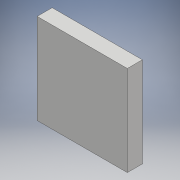
# Autodesk Inventor part: example_sample
Saved by Autodesk Inventor 2017 (Build 210142000, 142)
## iProperties
Created: 2018-01-08
Part Number: example_sample
Material: Generic
Document SubType Name: Modeling
Designer: Sam
Density: 1 g/cm^3
Appearance: Default
Author: Sam
Autodesk Inventor part; units mm, degrees
ref_plane "YZ Plane" through (0, 0, 0) normal (1, 0, 0) x (0, 1, 0)
ref_plane "XZ Plane" through (0, 0, 0) normal (0, 1, 0) x (-1, 0, 0)
ref_plane "XY Plane" through (0, 0, 0) normal (0, 0, 1) x (1, 0, 0)
sketch "Sketch1" plane through (0, 0, 0) normal (0, 1, 0) x (-1, 0, 0)
  line L0 (6, 6) -> (-6, 6)
  line L1 (-6, 6) -> (-6, -6)
  line L2 (-6, -6) -> (6, -6)
  line L3 (6, -6) -> (6, 6)
  line L4 (6, 6) -> (-6, -6) construction
  line L5 (-6, 6) -> (6, -6) construction
  point P0 (0, 0)
  dimension "d0" = 12
  dimension "d1" = 12
  constraints: 12 end point, 2 midpoint, 2 parallel, 1 horizontal, 1 perpendicular
  measures "d0" distance of L2.end L1.end
  measures "d1" distance of L1.end L0.end
extrude "Extrusion1" add sketch "Sketch1" along normal blind 2
sketch "Sketch2" plane through (0, 2, 0) normal (0, 1, 0) x (1, 0, 0)
  line L0 (-0.0927, -0.2032) -> (0.0511, -0.2032)
  line L1 (0.0511, -0.2032) -> (-0.1769, -0.0781)
  line L2 (-0.1769, -0.0781) -> (-0.1593, -0.3245)
  line L3 (-0.1593, -0.3245) -> (-0.0927, -0.2032)
  line L4 (-0.0811, 0.2563) -> (-0.126, 0.1039)
  line L5 (-0.126, 0.1039) -> (-0.0159, 0.0999)
  line L6 (-0.0159, 0.0999) -> (-0.0811, 0.2563)
  line L7 (0.315, -0.1506) -> (0.1499, 0.28)
  line L8 (0.1499, 0.28) -> (0.0261, 0.2325)
  line L9 (0.0261, 0.2325) -> (0.1912, -0.198)
  line L10 (0.1912, -0.198) -> (0.315, -0.1506)
  line L11 (0.315, -0.1506) -> (0.0261, 0.2325) construction
  line L12 (0.1499, 0.28) -> (0.1912, -0.198) construction
  point P0 (0, 0)
  point P1 (0.1705, 0.041)
  constraints: 26 end point, 2 midpoint, 2 parallel, 2 perpendicular, 1 horizontal
extrude "Extrusion2" cut sketch "Sketch2" along normal mid plane 0.06 contours L3 L2 L1 L0
extrude "Extrusion3" add sketch "Sketch2" along normal blind 0.03 contours L6 L5 L4
extrude "Extrusion4" add sketch "Sketch2" along normal blind 0.02 contours L10 L9 L8 L7
draft "FaceDraft1" angle 20 pull direction (-0.9337322, 0, 0.3579724) faces at (0.2187, 2.02, 0.0229) fixed edges at (0.1086, 2.02, -0.0173)
body "Solid1"
